Autodesk Fusion 360 part; units mm, degrees
(part 2 of 2)
  arc A221 (-17.6971, -6.491) -> (-17.5951, -6.2945) centre (-17.5563, -6.4394) cw
  arc A222 (-18.1326, 5.1508) -> (-17.9345, 5.2498) centre (-17.9883, 5.1098) cw
  arc A223 (-17.4949, -7.0179) -> (-17.6971, -6.491) centre (0, 0) cw
  arc A224 (-15.4345, -10.5349) -> (-15.6535, -10.5019) centre (-15.5289, -10.4184) cw
  arc A225 (-17.2875, 7.0957) -> (-16.8407, 8.0992) centre (-17.0376, 7.5856) ccw
  arc A226 (-16.9217, 8.3053) -> (-16.6655, 8.8082) centre (0, 0) cw
  arc A227 (-18.1566, -4.4208) -> (-18.385, -3.3464) centre (-18.2425, -3.8776) ccw
  arc A228 (-18.8368, -0.7046) -> (-18.679, -0.5492) centre (-18.6869, -0.699) cw
  arc A229 (-17.5951, 6.2945) -> (-17.6971, 6.491) centre (-17.5563, 6.4394) cw
  arc A230 (-17.9345, -5.2498) -> (-18.1326, -5.1508) centre (-17.9883, -5.1098) cw
  arc A231 (-18.1566, 4.4208) -> (-18.2787, 4.6056) centre (-18.1332, 4.569) cw
  arc A232 (-17.4949, 7.0179) -> (-17.2875, 7.0957) centre (-17.3557, 6.9621) cw
  arc A233 (-18.679, -0.5492) -> (-18.679, 0.5492) centre (-18.65, 0) ccw
  arc A234 (-14.2487, -12.0905) -> (-14.47, -12.0807) centre (-14.3548, -11.9845) cw
  arc A235 (-18.66, 2.6698) -> (-18.5717, 3.2272) centre (0, 0) cw
  arc A236 (-15.4345, 10.5349) -> (-14.7888, 11.4236) centre (-15.0882, 10.9622) ccw
  arc A237 (-15.9609, 10.0286) -> (-15.6535, 10.5019) centre (0, 0) cw
  arc A238 (-14.7888, 11.4236) -> (-14.8251, 11.6421) centre (-14.7072, 11.5494) cw
  arc A239 (-14.47, 12.0807) -> (-14.2487, 12.0905) centre (-14.3548, 11.9845) cw
  circle A240 centre (0, 0) radius 19
extrude "Extrude2" add sketch "60t gt2" along normal blind 7 contours A0 A1 A2 A3 A4 A5 A6 A7 A8 A9 A10 A11 A12 A13 A14 A15 A16 A17 A18 A19 A20 A21 A22 A23 A24 A25 A26 A27 A28 A29 A30 A31 A32 A33 A34 A35 A36 A37 A38 A39 A40 A41 A42 A43 A44 A45 A46 A47 A48 A49 A50 A51 A52 A53 A54 A55 A56 A57 A58 A59 A60 A61 A62 A63 A64 A65 A66 A67 A68 A69 A70 A71 A72 A73 A74 A75 A76 A77 A78 A79 A80 A81 A82 A83 A84 A85 A86 A87 A88 A89 A90 A91 A92 A93 A94 A95 A96 A97 A98 A99 A100 A101 A102 A103 A104 A105 A106 A107 A108 A109 A110 A111 A112 A113 A114 A115 A116 A117 A118 A119 A120 A121 A122 A123 A124 A125 A126 A127 A128 A129 A130 A131 A132 A133 A134 A135 A136 A137 A138 A139 A140 A141 A142 A143 A144 A145 A146 A147 A148 A149 A150 A151 A152 A153 A154 A155 A156 A157 A158 A159 A160 A161 A162 A163 A164 A165 A166 A167 A168 A169 A170 A171 A172 A173 A174 A175 A176 A177 A178 A179 A180 A181 A182 A183 A184 A185 A186 A187 A188 A189 A190 A191 A192 A193 A194 A195 A196 A197 A198 A199 A200 A201 A202 A203 A204 A205 A206 A207 A208 A209 A210 A211 A212 A213 A214 A215 A216 A217 A218 A219 A220 A221 A222 A223 A224 A225 A226 A227 A228 A229 A230 A231 A232 A233 A234 A235 A236 A237 A238 A239
sketch "Sketch8" plane through (0, 0, 0) normal (0, 0, -1) x (1, 0, 0)
  circle A0 centre (0, 0) radius 20
  arc A1 (-14.8251, -11.6421) -> (-14.47, -12.0807) centre (0, 0) ccw
  arc A2 (-14.47, -12.0807) -> (-14.2487, -12.0905) centre (-14.3548, -11.9845) ccw
  arc A3 (-13.5137, -12.9069) -> (-14.2487, -12.0905) centre (-13.8597, -12.4793) ccw
  arc A4 (-13.5137, -12.9069) -> (-13.527, -13.1279) centre (-13.4194, -13.0235) ccw
  arc A5 (-13.527, -13.1279) -> (-13.1279, -13.527) centre (0, 0) ccw
  arc A6 (-13.1279, -13.527) -> (-12.9069, -13.5137) centre (-13.0235, -13.4194) ccw
  arc A7 (-12.0905, -14.2487) -> (-12.9069, -13.5137) centre (-12.4793, -13.8597) ccw
  arc A8 (-12.0905, -14.2487) -> (-12.0807, -14.47) centre (-11.9845, -14.3548) ccw
  arc A9 (-12.0807, -14.47) -> (-11.6421, -14.8251) centre (0, 0) ccw
  arc A10 (-11.6421, -14.8251) -> (-11.4236, -14.7888) centre (-11.5494, -14.7072) ccw
  arc A11 (-10.5349, -15.4345) -> (-11.4236, -14.7888) centre (-10.9622, -15.0882) ccw
  arc A12 (-10.5349, -15.4345) -> (-10.5019, -15.6535) centre (-10.4184, -15.5289) ccw
  arc A13 (-10.5019, -15.6535) -> (-10.0286, -15.9609) centre (0, 0) ccw
  arc A14 (-10.0286, -15.9609) -> (-9.8152, -15.9019) centre (-9.9488, -15.8338) ccw
  arc A15 (-8.8639, -16.4511) -> (-9.8152, -15.9019) centre (-9.325, -16.1514) ccw
  arc A16 (-8.8639, -16.4511) -> (-8.8082, -16.6655) centre (-8.7381, -16.5329) ccw
  arc A17 (-8.8082, -16.6655) -> (-8.3053, -16.9217) centre (0, 0) ccw
  arc A18 (-8.3053, -16.9217) -> (-8.0992, -16.8407) centre (-8.2393, -16.787) ccw
  arc A19 (-7.0957, -17.2875) -> (-8.0992, -16.8407) centre (-7.5856, -17.0376) ccw
  arc A20 (-7.0957, -17.2875) -> (-7.0179, -17.4949) centre (-6.9621, -17.3557) ccw
  arc A21 (-7.0179, -17.4949) -> (-6.491, -17.6971) centre (0, 0) ccw
  arc A22 (-6.491, -17.6971) -> (-6.2945, -17.5951) centre (-6.4394, -17.5563) ccw
  arc A23 (-5.2498, -17.9345) -> (-6.2945, -17.5951) centre (-5.7632, -17.7372) ccw
  arc A24 (-5.2498, -17.9345) -> (-5.1508, -18.1326) centre (-5.1098, -17.9883) ccw
  arc A25 (-5.1508, -18.1326) -> (-4.6056, -18.2787) centre (0, 0) ccw
  arc A26 (-4.6056, -18.2787) -> (-4.4208, -18.1566) centre (-4.569, -18.1332) ccw
  arc A27 (-3.3464, -18.385) -> (-4.4208, -18.1566) centre (-3.8776, -18.2425) ccw
  arc A28 (-3.3464, -18.385) -> (-3.2272, -18.5717) centre (-3.2015, -18.4239) ccw
  arc A29 (-3.2272, -18.5717) -> (-2.6698, -18.66) centre (0, 0) ccw
  arc A30 (-2.6698, -18.66) -> (-2.4987, -18.5193) centre (-2.6485, -18.5115) ccw
  arc A31 (-1.4063, -18.6341) -> (-2.4987, -18.5193) centre (-1.9495, -18.5478) ccw
  arc A32 (-1.4063, -18.6341) -> (-1.2682, -18.8073) centre (-1.2581, -18.6576) ccw
  arc A33 (-1.2682, -18.8073) -> (-0.7046, -18.8368) centre (0, 0) ccw
  arc A34 (-0.7046, -18.8368) -> (-0.5492, -18.679) centre (-0.699, -18.6869) ccw
  arc A35 (0.5492, -18.679) -> (-0.5492, -18.679) centre (0, -18.65) ccw
  arc A36 (0.5492, -18.679) -> (0.7046, -18.8368) centre (0.699, -18.6869) ccw
  arc A37 (0.7046, -18.8368) -> (1.2682, -18.8073) centre (0, 0) ccw
  arc A38 (1.2682, -18.8073) -> (1.4063, -18.6341) centre (1.2581, -18.6576) ccw
  arc A39 (2.4987, -18.5193) -> (1.4063, -18.6341) centre (1.9495, -18.5478) ccw
  arc A40 (2.4987, -18.5193) -> (2.6698, -18.66) centre (2.6485, -18.5115) ccw
  arc A41 (2.6698, -18.66) -> (3.2272, -18.5717) centre (0, 0) ccw
  arc A42 (3.2272, -18.5717) -> (3.3464, -18.385) centre (3.2015, -18.4239) ccw
  arc A43 (4.4208, -18.1566) -> (3.3464, -18.385) centre (3.8776, -18.2425) ccw
  arc A44 (4.4208, -18.1566) -> (4.6056, -18.2787) centre (4.569, -18.1332) ccw
  arc A45 (4.6056, -18.2787) -> (5.1508, -18.1326) centre (0, 0) ccw
  arc A46 (5.1508, -18.1326) -> (5.2498, -17.9345) centre (5.1098, -17.9883) ccw
  arc A47 (6.2945, -17.5951) -> (5.2498, -17.9345) centre (5.7632, -17.7372) ccw
  arc A48 (6.2945, -17.5951) -> (6.491, -17.6971) centre (6.4394, -17.5563) ccw
  arc A49 (6.491, -17.6971) -> (7.0179, -17.4949) centre (0, 0) ccw
  arc A50 (7.0179, -17.4949) -> (7.0957, -17.2875) centre (6.9621, -17.3557) ccw
  arc A51 (8.0992, -16.8407) -> (7.0957, -17.2875) centre (7.5856, -17.0376) ccw
  arc A52 (8.0992, -16.8407) -> (8.3053, -16.9217) centre (8.2393, -16.787) ccw
  arc A53 (8.3053, -16.9217) -> (8.8082, -16.6655) centre (0, 0) ccw
  arc A54 (8.8082, -16.6655) -> (8.8639, -16.4511) centre (8.7381, -16.5329) ccw
  arc A55 (9.8152, -15.9019) -> (8.8639, -16.4511) centre (9.325, -16.1514) ccw
  arc A56 (9.8152, -15.9019) -> (10.0286, -15.9609) centre (9.9488, -15.8338) ccw
  arc A57 (10.0286, -15.9609) -> (10.5019, -15.6535) centre (0, 0) ccw
  arc A58 (10.5019, -15.6535) -> (10.5349, -15.4345) centre (10.4184, -15.5289) ccw
  arc A59 (11.4236, -14.7888) -> (10.5349, -15.4345) centre (10.9622, -15.0882) ccw
  arc A60 (11.4236, -14.7888) -> (11.6421, -14.8251) centre (11.5494, -14.7072) ccw
  arc A61 (11.6421, -14.8251) -> (12.0807, -14.47) centre (0, 0) ccw
  arc A62 (12.0807, -14.47) -> (12.0905, -14.2487) centre (11.9845, -14.3548) ccw
  arc A63 (12.9069, -13.5137) -> (12.0905, -14.2487) centre (12.4793, -13.8597) ccw
  arc A64 (12.9069, -13.5137) -> (13.1279, -13.527) centre (13.0235, -13.4194) ccw
  arc A65 (13.1279, -13.527) -> (13.527, -13.1279) centre (0, 0) ccw
  arc A66 (13.527, -13.1279) -> (13.5137, -12.9069) centre (13.4194, -13.0235) ccw
  arc A67 (14.2487, -12.0905) -> (13.5137, -12.9069) centre (13.8597, -12.4793) ccw
  arc A68 (14.2487, -12.0905) -> (14.47, -12.0807) centre (14.3548, -11.9845) ccw
  arc A69 (14.47, -12.0807) -> (14.8251, -11.6421) centre (0, 0) ccw
  arc A70 (14.8251, -11.6421) -> (14.7888, -11.4236) centre (14.7072, -11.5494) ccw
  arc A71 (15.4345, -10.5349) -> (14.7888, -11.4236) centre (15.0882, -10.9622) ccw
  arc A72 (15.4345, -10.5349) -> (15.6535, -10.5019) centre (15.5289, -10.4184) ccw
  arc A73 (15.6535, -10.5019) -> (15.9609, -10.0286) centre (0, 0) ccw
  arc A74 (15.9609, -10.0286) -> (15.9019, -9.8152) centre (15.8338, -9.9488) ccw
  arc A75 (16.4511, -8.8639) -> (15.9019, -9.8152) centre (16.1514, -9.325) ccw
  arc A76 (16.4511, -8.8639) -> (16.6655, -8.8082) centre (16.5329, -8.7381) ccw
  arc A77 (16.6655, -8.8082) -> (16.9217, -8.3053) centre (0, 0) ccw
  arc A78 (16.9217, -8.3053) -> (16.8407, -8.0992) centre (16.787, -8.2393) ccw
  arc A79 (17.2875, -7.0957) -> (16.8407, -8.0992) centre (17.0376, -7.5856) ccw
  arc A80 (17.2875, -7.0957) -> (17.4949, -7.0179) centre (17.3557, -6.9621) ccw
  arc A81 (17.4949, -7.0179) -> (17.6971, -6.491) centre (0, 0) ccw
  arc A82 (17.6971, -6.491) -> (17.5951, -6.2945) centre (17.5563, -6.4394) ccw
  arc A83 (17.9345, -5.2498) -> (17.5951, -6.2945) centre (17.7372, -5.7632) ccw
  arc A84 (17.9345, -5.2498) -> (18.1326, -5.1508) centre (17.9883, -5.1098) ccw
  arc A85 (18.1326, -5.1508) -> (18.2787, -4.6056) centre (0, 0) ccw
  arc A86 (18.2787, -4.6056) -> (18.1566, -4.4208) centre (18.1332, -4.569) ccw
  arc A87 (18.385, -3.3464) -> (18.1566, -4.4208) centre (18.2425, -3.8776) ccw
  arc A88 (18.385, -3.3464) -> (18.5717, -3.2272) centre (18.4239, -3.2015) ccw
  arc A89 (18.5717, -3.2272) -> (18.66, -2.6698) centre (0, 0) ccw
  arc A90 (18.66, -2.6698) -> (18.5193, -2.4987) centre (18.5115, -2.6485) ccw
  arc A91 (18.6341, -1.4063) -> (18.5193, -2.4987) centre (18.5478, -1.9495) ccw
  arc A92 (18.6341, -1.4063) -> (18.8073, -1.2682) centre (18.6576, -1.2581) ccw
  arc A93 (18.8073, -1.2682) -> (18.8368, -0.7046) centre (0, 0) ccw
  arc A94 (18.8368, -0.7046) -> (18.679, -0.5492) centre (18.6869, -0.699) ccw
  arc A95 (18.679, 0.5492) -> (18.679, -0.5492) centre (18.65, 0) ccw
  arc A96 (18.679, 0.5492) -> (18.8368, 0.7046) centre (18.6869, 0.699) ccw
  arc A97 (18.8368, 0.7046) -> (18.8073, 1.2682) centre (0, 0) ccw
  arc A98 (18.8073, 1.2682) -> (18.6341, 1.4063) centre (18.6576, 1.2581) ccw
  arc A99 (18.5193, 2.4987) -> (18.6341, 1.4063) centre (18.5478, 1.9495) ccw
  arc A100 (18.5193, 2.4987) -> (18.66, 2.6698) centre (18.5115, 2.6485) ccw
  arc A101 (18.66, 2.6698) -> (18.5717, 3.2272) centre (0, 0) ccw
  arc A102 (18.5717, 3.2272) -> (18.385, 3.3464) centre (18.4239, 3.2015) ccw
  arc A103 (18.1566, 4.4208) -> (18.385, 3.3464) centre (18.2425, 3.8776) ccw
  arc A104 (18.1566, 4.4208) -> (18.2787, 4.6056) centre (18.1332, 4.569) ccw
  arc A105 (18.2787, 4.6056) -> (18.1326, 5.1508) centre (0, 0) ccw
  arc A106 (18.1326, 5.1508) -> (17.9345, 5.2498) centre (17.9883, 5.1098) ccw
  arc A107 (17.5951, 6.2945) -> (17.9345, 5.2498) centre (17.7372, 5.7632) ccw
  arc A108 (17.5951, 6.2945) -> (17.6971, 6.491) centre (17.5563, 6.4394) ccw
  arc A109 (17.6971, 6.491) -> (17.4949, 7.0179) centre (0, 0) ccw
  arc A110 (17.4949, 7.0179) -> (17.2875, 7.0957) centre (17.3557, 6.9621) ccw
  arc A111 (16.8407, 8.0992) -> (17.2875, 7.0957) centre (17.0376, 7.5856) ccw
  arc A112 (16.8407, 8.0992) -> (16.9217, 8.3053) centre (16.787, 8.2393) ccw
  arc A113 (16.9217, 8.3053) -> (16.6655, 8.8082) centre (0, 0) ccw
  arc A114 (16.6655, 8.8082) -> (16.4511, 8.8639) centre (16.5329, 8.7381) ccw
  arc A115 (15.9019, 9.8152) -> (16.4511, 8.8639) centre (16.1514, 9.325) ccw
  arc A116 (15.9019, 9.8152) -> (15.9609, 10.0286) centre (15.8338, 9.9488) ccw
  arc A117 (15.9609, 10.0286) -> (15.6535, 10.5019) centre (0, 0) ccw
  arc A118 (15.6535, 10.5019) -> (15.4345, 10.5349) centre (15.5289, 10.4184) ccw
  arc A119 (14.7888, 11.4236) -> (15.4345, 10.5349) centre (15.0882, 10.9622) ccw
  arc A120 (14.7888, 11.4236) -> (14.8251, 11.6421) centre (14.7072, 11.5494) ccw
  arc A121 (14.8251, 11.6421) -> (14.47, 12.0807) centre (0, 0) ccw
  arc A122 (14.47, 12.0807) -> (14.2487, 12.0905) centre (14.3548, 11.9845) ccw
  arc A123 (13.5137, 12.9069) -> (14.2487, 12.0905) centre (13.8597, 12.4793) ccw
  arc A124 (13.5137, 12.9069) -> (13.527, 13.1279) centre (13.4194, 13.0235) ccw
  arc A125 (13.527, 13.1279) -> (13.1279, 13.527) centre (0, 0) ccw
  arc A126 (13.1279, 13.527) -> (12.9069, 13.5137) centre (13.0235, 13.4194) ccw
  arc A127 (12.0905, 14.2487) -> (12.9069, 13.5137) centre (12.4793, 13.8597) ccw
  arc A128 (12.0905, 14.2487) -> (12.0807, 14.47) centre (11.9845, 14.3548) ccw
  arc A129 (12.0807, 14.47) -> (11.6421, 14.8251) centre (0, 0) ccw
  arc A130 (11.6421, 14.8251) -> (11.4236, 14.7888) centre (11.5494, 14.7072) ccw
  arc A131 (10.5349, 15.4345) -> (11.4236, 14.7888) centre (10.9622, 15.0882) ccw
  arc A132 (10.5349, 15.4345) -> (10.5019, 15.6535) centre (10.4184, 15.5289) ccw
  arc A133 (10.5019, 15.6535) -> (10.0286, 15.9609) centre (0, 0) ccw
  arc A134 (10.0286, 15.9609) -> (9.8152, 15.9019) centre (9.9488, 15.8338) ccw
  arc A135 (8.8639, 16.4511) -> (9.8152, 15.9019) centre (9.325, 16.1514) ccw
  arc A136 (8.8639, 16.4511) -> (8.8082, 16.6655) centre (8.7381, 16.5329) ccw
  arc A137 (8.8082, 16.6655) -> (8.3053, 16.9217) centre (0, 0) ccw
  arc A138 (8.3053, 16.9217) -> (8.0992, 16.8407) centre (8.2393, 16.787) ccw
  arc A139 (7.0957, 17.2875) -> (8.0992, 16.8407) centre (7.5856, 17.0376) ccw
  arc A140 (7.0957, 17.2875) -> (7.0179, 17.4949) centre (6.9621, 17.3557) ccw
  arc A141 (7.0179, 17.4949) -> (6.491, 17.6971) centre (0, 0) ccw
  arc A142 (6.491, 17.6971) -> (6.2945, 17.5951) centre (6.4394, 17.5563) ccw
  arc A143 (5.2498, 17.9345) -> (6.2945, 17.5951) centre (5.7632, 17.7372) ccw
  arc A144 (5.2498, 17.9345) -> (5.1508, 18.1326) centre (5.1098, 17.9883) ccw
  arc A145 (5.1508, 18.1326) -> (4.6056, 18.2787) centre (0, 0) ccw
  arc A146 (4.6056, 18.2787) -> (4.4208, 18.1566) centre (4.569, 18.1332) ccw
  arc A147 (3.3464, 18.385) -> (4.4208, 18.1566) centre (3.8776, 18.2425) ccw
  arc A148 (3.3464, 18.385) -> (3.2272, 18.5717) centre (3.2015, 18.4239) ccw
  arc A149 (3.2272, 18.5717) -> (2.6698, 18.66) centre (0, 0) ccw
  arc A150 (2.6698, 18.66) -> (2.4987, 18.5193) centre (2.6485, 18.5115) ccw
  arc A151 (1.4063, 18.6341) -> (2.4987, 18.5193) centre (1.9495, 18.5478) ccw
  arc A152 (1.4063, 18.6341) -> (1.2682, 18.8073) centre (1.2581, 18.6576) ccw
  arc A153 (1.2682, 18.8073) -> (0.7046, 18.8368) centre (0, 0) ccw
  arc A154 (0.7046, 18.8368) -> (0.5492, 18.679) centre (0.699, 18.6869) ccw
  arc A155 (-0.5492, 18.679) -> (0.5492, 18.679) centre (0, 18.65) ccw
  arc A156 (-0.5492, 18.679) -> (-0.7046, 18.8368) centre (-0.699, 18.6869) ccw
  arc A157 (-0.7046, 18.8368) -> (-1.2682, 18.8073) centre (0, 0) ccw
  arc A158 (-1.2682, 18.8073) -> (-1.4063, 18.6341) centre (-1.2581, 18.6576) ccw
  arc A159 (-2.4987, 18.5193) -> (-1.4063, 18.6341) centre (-1.9495, 18.5478) ccw
  arc A160 (-2.4987, 18.5193) -> (-2.6698, 18.66) centre (-2.6485, 18.5115) ccw
  arc A161 (-2.6698, 18.66) -> (-3.2272, 18.5717) centre (0, 0) ccw
  arc A162 (-3.2272, 18.5717) -> (-3.3464, 18.385) centre (-3.2015, 18.4239) ccw
  arc A163 (-4.4208, 18.1566) -> (-3.3464, 18.385) centre (-3.8776, 18.2425) ccw
  arc A164 (-4.4208, 18.1566) -> (-4.6056, 18.2787) centre (-4.569, 18.1332) ccw
  arc A165 (-4.6056, 18.2787) -> (-5.1508, 18.1326) centre (0, 0) ccw
  arc A166 (-5.1508, 18.1326) -> (-5.2498, 17.9345) centre (-5.1098, 17.9883) ccw
  arc A167 (-6.2945, 17.5951) -> (-5.2498, 17.9345) centre (-5.7632, 17.7372) ccw
  arc A168 (-6.2945, 17.5951) -> (-6.491, 17.6971) centre (-6.4394, 17.5563) ccw
  arc A169 (-6.491, 17.6971) -> (-7.0179, 17.4949) centre (0, 0) ccw
  arc A170 (-7.0179, 17.4949) -> (-7.0957, 17.2875) centre (-6.9621, 17.3557) ccw
  arc A171 (-8.0992, 16.8407) -> (-7.0957, 17.2875) centre (-7.5856, 17.0376) ccw
  arc A172 (-8.0992, 16.8407) -> (-8.3053, 16.9217) centre (-8.2393, 16.787) ccw
  arc A173 (-8.3053, 16.9217) -> (-8.8082, 16.6655) centre (0, 0) ccw
  arc A174 (-8.8082, 16.6655) -> (-8.8639, 16.4511) centre (-8.7381, 16.5329) ccw
  arc A175 (-9.8152, 15.9019) -> (-8.8639, 16.4511) centre (-9.325, 16.1514) ccw
  arc A176 (-9.8152, 15.9019) -> (-10.0286, 15.9609) centre (-9.9488, 15.8338) ccw
  arc A177 (-10.0286, 15.9609) -> (-10.5019, 15.6535) centre (0, 0) ccw
  arc A178 (-10.5019, 15.6535) -> (-10.5349, 15.4345) centre (-10.4184, 15.5289) ccw
  arc A179 (-11.4236, 14.7888) -> (-10.5349, 15.4345) centre (-10.9622, 15.0882) ccw
  arc A180 (-11.4236, 14.7888) -> (-11.6421, 14.8251) centre (-11.5494, 14.7072) ccw
  arc A181 (-11.6421, 14.8251) -> (-12.0807, 14.47) centre (0, 0) ccw
  arc A182 (-12.0807, 14.47) -> (-12.0905, 14.2487) centre (-11.9845, 14.3548) ccw
  arc A183 (-12.9069, 13.5137) -> (-12.0905, 14.2487) centre (-12.4793, 13.8597) ccw
  arc A184 (-12.9069, 13.5137) -> (-13.1279, 13.527) centre (-13.0235, 13.4194) ccw
  arc A185 (-13.1279, 13.527) -> (-13.527, 13.1279) centre (0, 0) ccw
  arc A186 (-13.527, 13.1279) -> (-13.5137, 12.9069) centre (-13.4194, 13.0235) ccw
  arc A187 (-14.2487, 12.0905) -> (-13.5137, 12.9069) centre (-13.8597, 12.4793) ccw
  arc A188 (-14.2487, 12.0905) -> (-14.47, 12.0807) centre (-14.3548, 11.9845) ccw
  arc A189 (-14.47, 12.0807) -> (-14.8251, 11.6421) centre (0, 0) ccw
  arc A190 (-14.8251, 11.6421) -> (-14.7888, 11.4236) centre (-14.7072, 11.5494) ccw
  arc A191 (-15.4345, 10.5349) -> (-14.7888, 11.4236) centre (-15.0882, 10.9622) ccw
  arc A192 (-15.4345, 10.5349) -> (-15.6535, 10.5019) centre (-15.5289, 10.4184) ccw
  arc A193 (-15.6535, 10.5019) -> (-15.9609, 10.0286) centre (0, 0) ccw
  arc A194 (-15.9609, 10.0286) -> (-15.9019, 9.8152) centre (-15.8338, 9.9488) ccw
  arc A195 (-16.4511, 8.8639) -> (-15.9019, 9.8152) centre (-16.1514, 9.325) ccw
  arc A196 (-16.4511, 8.8639) -> (-16.6655, 8.8082) centre (-16.5329, 8.7381) ccw
  arc A197 (-16.6655, 8.8082) -> (-16.9217, 8.3053) centre (0, 0) ccw
  arc A198 (-16.9217, 8.3053) -> (-16.8407, 8.0992) centre (-16.787, 8.2393) ccw
  arc A199 (-17.2875, 7.0957) -> (-16.8407, 8.0992) centre (-17.0376, 7.5856) ccw
  arc A200 (-17.2875, 7.0957) -> (-17.4949, 7.0179) centre (-17.3557, 6.9621) ccw
  arc A201 (-17.4949, 7.0179) -> (-17.6971, 6.491) centre (0, 0) ccw
  arc A202 (-17.6971, 6.491) -> (-17.5951, 6.2945) centre (-17.5563, 6.4394) ccw
  arc A203 (-17.9345, 5.2498) -> (-17.5951, 6.2945) centre (-17.7372, 5.7632) ccw
  arc A204 (-17.9345, 5.2498) -> (-18.1326, 5.1508) centre (-17.9883, 5.1098) ccw
  arc A205 (-18.1326, 5.1508) -> (-18.2787, 4.6056) centre (0, 0) ccw
  arc A206 (-18.2787, 4.6056) -> (-18.1566, 4.4208) centre (-18.1332, 4.569) ccw
  arc A207 (-18.385, 3.3464) -> (-18.1566, 4.4208) centre (-18.2425, 3.8776) ccw
  arc A208 (-18.385, 3.3464) -> (-18.5717, 3.2272) centre (-18.4239, 3.2015) ccw
  arc A209 (-18.5717, 3.2272) -> (-18.66, 2.6698) centre (0, 0) ccw
  arc A210 (-18.66, 2.6698) -> (-18.5193, 2.4987) centre (-18.5115, 2.6485) ccw
  arc A211 (-18.6341, 1.4063) -> (-18.5193, 2.4987) centre (-18.5478, 1.9495) ccw
  arc A212 (-18.6341, 1.4063) -> (-18.8073, 1.2682) centre (-18.6576, 1.2581) ccw
  arc A213 (-18.8073, 1.2682) -> (-18.8368, 0.7046) centre (0, 0) ccw
  arc A214 (-18.8368, 0.7046) -> (-18.679, 0.5492) centre (-18.6869, 0.699) ccw
  arc A215 (-18.679, -0.5492) -> (-18.679, 0.5492) centre (-18.65, 0) ccw
  arc A216 (-18.679, -0.5492) -> (-18.8368, -0.7046) centre (-18.6869, -0.699) ccw
  arc A217 (-18.8368, -0.7046) -> (-18.8073, -1.2682) centre (0, 0) ccw
  arc A218 (-18.8073, -1.2682) -> (-18.6341, -1.4063) centre (-18.6576, -1.2581) ccw
  arc A219 (-18.5193, -2.4987) -> (-18.6341, -1.4063) centre (-18.5478, -1.9495) ccw
  arc A220 (-18.5193, -2.4987) -> (-18.66, -2.6698) centre (-18.5115, -2.6485) ccw
  arc A221 (-18.66, -2.6698) -> (-18.5717, -3.2272) centre (0, 0) ccw
  arc A222 (-18.5717, -3.2272) -> (-18.385, -3.3464) centre (-18.4239, -3.2015) ccw
  arc A223 (-18.1566, -4.4208) -> (-18.385, -3.3464) centre (-18.2425, -3.8776) ccw
  arc A224 (-18.1566, -4.4208) -> (-18.2787, -4.6056) centre (-18.1332, -4.569) ccw
  arc A225 (-18.2787, -4.6056) -> (-18.1326, -5.1508) centre (0, 0) ccw
  arc A226 (-18.1326, -5.1508) -> (-17.9345, -5.2498) centre (-17.9883, -5.1098) ccw
  arc A227 (-17.5951, -6.2945) -> (-17.9345, -5.2498) centre (-17.7372, -5.7632) ccw
  arc A228 (-17.5951, -6.2945) -> (-17.6971, -6.491) centre (-17.5563, -6.4394) ccw
  arc A229 (-17.6971, -6.491) -> (-17.4949, -7.0179) centre (0, 0) ccw
  arc A230 (-17.4949, -7.0179) -> (-17.2875, -7.0957) centre (-17.3557, -6.9621) ccw
  arc A231 (-16.8407, -8.0992) -> (-17.2875, -7.0957) centre (-17.0376, -7.5856) ccw
  arc A232 (-16.8407, -8.0992) -> (-16.9217, -8.3053) centre (-16.787, -8.2393) ccw
  arc A233 (-16.9217, -8.3053) -> (-16.6655, -8.8082) centre (0, 0) ccw
  arc A234 (-16.6655, -8.8082) -> (-16.4511, -8.8639) centre (-16.5329, -8.7381) ccw
  arc A235 (-15.9019, -9.8152) -> (-16.4511, -8.8639) centre (-16.1514, -9.325) ccw
  arc A236 (-15.9019, -9.8152) -> (-15.9609, -10.0286) centre (-15.8338, -9.9488) ccw
  arc A237 (-15.9609, -10.0286) -> (-15.6535, -10.5019) centre (0, 0) ccw
  arc A238 (-15.6535, -10.5019) -> (-15.4345, -10.5349) centre (-15.5289, -10.4184) ccw
  arc A239 (-14.7888, -11.4236) -> (-15.4345, -10.5349) centre (-15.0882, -10.9622) ccw
  arc A240 (-14.7888, -11.4236) -> (-14.8251, -11.6421) centre (-14.7072, -11.5494) ccw
  dimension "d55" = 40
  constraint coincident A0.centre A1.centre
  measures "d55" diameter of A0
extrude "Extrude9" add sketch "Sketch8" along normal blind 1 contours A0 | A1 A2 A3 A4 A5 A6 A7 A8 A9 A10 A11 A12 A13 A14 A15 A16 A17 A18 A19 A20 A21 A22 A23 A24 A25 A26 A27 A28 A29 A30 A31 A32 A33 A34 A35 A36 A37 A38 A39 A40 A41 A42 A43 A44 A45 A46 A47 A48 A49 A50 A51 A52 A53 A54 A55 A56 A57 A58 A59 A60 A61 A62 A63 A64 A65 A66 A67 A68 A69 A70 A71 A72 A73 A74 A75 A76 A77 A78 A79 A80 A81 A82 A83 A84 A85 A86 A87 A88 A89 A90 A91 A92 A93 A94 A95 A96 A97 A98 A99 A100 A101 A102 A103 A104 A105 A106 A107 A108 A109 A110 A111 A112 A113 A114 A115 A116 A117 A118 A119 A120 A121 A122 A123 A124 A125 A126 A127 A128 A129 A130 A131 A132 A133 A134 A135 A136 A137 A138 A139 A140 A141 A142 A143 A144 A145 A146 A147 A148 A149 A150 A151 A152 A153 A154 A155 A156 A157 A158 A159 A160 A161 A162 A163 A164 A165 A166 A167 A168 A169 A170 A171 A172 A173 A174 A175 A176 A177 A178 A179 A180 A181 A182 A183 A184 A185 A186 A187 A188 A189 A190 A191 A192 A193 A194 A195 A196 A197 A198 A199 A200 A201 A202 A203 A204 A205 A206 A207 A208 A209 A210 A211 A212 A213 A214 A215 A216 A217 A218 A219 A220 A221 A222 A223 A224 A225 A226 A227 A228 A229 A230 A231 A232 A233 A234 A235 A236 A237 A238 A239 A240
sketch "Sketch9" plane through (0, 0, 7) normal (0, 0, 1) x (-1, 0, 0)
  circle A0 centre (0, 0) radius 20
  arc A1 (14.47, -12.0807) -> (14.8251, -11.6421) centre (0, 0) ccw
  arc A2 (14.8251, -11.6421) -> (14.7888, -11.4236) centre (14.7072, -11.5494) ccw
  arc A3 (15.4345, -10.5349) -> (14.7888, -11.4236) centre (15.0882, -10.9622) ccw
  arc A4 (15.4345, -10.5349) -> (15.6535, -10.5019) centre (15.5289, -10.4184) ccw
  arc A5 (15.6535, -10.5019) -> (15.9609, -10.0286) centre (0, 0) ccw
  arc A6 (15.9609, -10.0286) -> (15.9019, -9.8152) centre (15.8338, -9.9488) ccw
  arc A7 (16.4511, -8.8639) -> (15.9019, -9.8152) centre (16.1514, -9.325) ccw
  arc A8 (16.4511, -8.8639) -> (16.6655, -8.8082) centre (16.5329, -8.7381) ccw
  arc A9 (16.6655, -8.8082) -> (16.9217, -8.3053) centre (0, 0) ccw
  arc A10 (16.9217, -8.3053) -> (16.8407, -8.0992) centre (16.787, -8.2393) ccw
  arc A11 (17.2875, -7.0957) -> (16.8407, -8.0992) centre (17.0376, -7.5856) ccw
  arc A12 (17.2875, -7.0957) -> (17.4949, -7.0179) centre (17.3557, -6.9621) ccw
  arc A13 (17.4949, -7.0179) -> (17.6971, -6.491) centre (0, 0) ccw
  arc A14 (17.6971, -6.491) -> (17.5951, -6.2945) centre (17.5563, -6.4394) ccw
  arc A15 (17.9345, -5.2498) -> (17.5951, -6.2945) centre (17.7372, -5.7632) ccw
  arc A16 (17.9345, -5.2498) -> (18.1326, -5.1508) centre (17.9883, -5.1098) ccw
  arc A17 (18.1326, -5.1508) -> (18.2787, -4.6056) centre (0, 0) ccw
  arc A18 (18.2787, -4.6056) -> (18.1566, -4.4208) centre (18.1332, -4.569) ccw
  arc A19 (18.385, -3.3464) -> (18.1566, -4.4208) centre (18.2425, -3.8776) ccw
  arc A20 (18.385, -3.3464) -> (18.5717, -3.2272) centre (18.4239, -3.2015) ccw
  arc A21 (18.5717, -3.2272) -> (18.66, -2.6698) centre (0, 0) ccw
  arc A22 (18.66, -2.6698) -> (18.5193, -2.4987) centre (18.5115, -2.6485) ccw
  arc A23 (18.6341, -1.4063) -> (18.5193, -2.4987) centre (18.5478, -1.9495) ccw
  arc A24 (18.6341, -1.4063) -> (18.8073, -1.2682) centre (18.6576, -1.2581) ccw
  arc A25 (18.8073, -1.2682) -> (18.8368, -0.7046) centre (0, 0) ccw
  arc A26 (18.8368, -0.7046) -> (18.679, -0.5492) centre (18.6869, -0.699) ccw
  arc A27 (18.679, 0.5492) -> (18.679, -0.5492) centre (18.65, 0) ccw
  arc A28 (18.679, 0.5492) -> (18.8368, 0.7046) centre (18.6869, 0.699) ccw
  arc A29 (18.8368, 0.7046) -> (18.8073, 1.2682) centre (0, 0) ccw
  arc A30 (18.8073, 1.2682) -> (18.6341, 1.4063) centre (18.6576, 1.2581) ccw
  arc A31 (18.5193, 2.4987) -> (18.6341, 1.4063) centre (18.5478, 1.9495) ccw
  arc A32 (18.5193, 2.4987) -> (18.66, 2.6698) centre (18.5115, 2.6485) ccw
  arc A33 (18.66, 2.6698) -> (18.5717, 3.2272) centre (0, 0) ccw
  arc A34 (18.5717, 3.2272) -> (18.385, 3.3464) centre (18.4239, 3.2015) ccw
  arc A35 (18.1566, 4.4208) -> (18.385, 3.3464) centre (18.2425, 3.8776) ccw
  arc A36 (18.1566, 4.4208) -> (18.2787, 4.6056) centre (18.1332, 4.569) ccw
  arc A37 (18.2787, 4.6056) -> (18.1326, 5.1508) centre (0, 0) ccw
  arc A38 (18.1326, 5.1508) -> (17.9345, 5.2498) centre (17.9883, 5.1098) ccw
  arc A39 (17.5951, 6.2945) -> (17.9345, 5.2498) centre (17.7372, 5.7632) ccw
  arc A40 (17.5951, 6.2945) -> (17.6971, 6.491) centre (17.5563, 6.4394) ccw
  arc A41 (17.6971, 6.491) -> (17.4949, 7.0179) centre (0, 0) ccw
  arc A42 (17.4949, 7.0179) -> (17.2875, 7.0957) centre (17.3557, 6.9621) ccw
  arc A43 (16.8407, 8.0992) -> (17.2875, 7.0957) centre (17.0376, 7.5856) ccw
  arc A44 (16.8407, 8.0992) -> (16.9217, 8.3053) centre (16.787, 8.2393) ccw
  arc A45 (16.9217, 8.3053) -> (16.6655, 8.8082) centre (0, 0) ccw
  arc A46 (16.6655, 8.8082) -> (16.4511, 8.8639) centre (16.5329, 8.7381) ccw
  arc A47 (15.9019, 9.8152) -> (16.4511, 8.8639) centre (16.1514, 9.325) ccw
  arc A48 (15.9019, 9.8152) -> (15.9609, 10.0286) centre (15.8338, 9.9488) ccw
  arc A49 (15.9609, 10.0286) -> (15.6535, 10.5019) centre (0, 0) ccw
  arc A50 (15.6535, 10.5019) -> (15.4345, 10.5349) centre (15.5289, 10.4184) ccw
  arc A51 (14.7888, 11.4236) -> (15.4345, 10.5349) centre (15.0882, 10.9622) ccw
  arc A52 (14.7888, 11.4236) -> (14.8251, 11.6421) centre (14.7072, 11.5494) ccw
  arc A53 (14.8251, 11.6421) -> (14.47, 12.0807) centre (0, 0) ccw
  arc A54 (14.47, 12.0807) -> (14.2487, 12.0905) centre (14.3548, 11.9845) ccw
  arc A55 (13.5137, 12.9069) -> (14.2487, 12.0905) centre (13.8597, 12.4793) ccw
  arc A56 (13.5137, 12.9069) -> (13.527, 13.1279) centre (13.4194, 13.0235) ccw
  arc A57 (13.527, 13.1279) -> (13.1279, 13.527) centre (0, 0) ccw
  arc A58 (13.1279, 13.527) -> (12.9069, 13.5137) centre (13.0235, 13.4194) ccw
  arc A59 (12.0905, 14.2487) -> (12.9069, 13.5137) centre (12.4793, 13.8597) ccw
  arc A60 (12.0905, 14.2487) -> (12.0807, 14.47) centre (11.9845, 14.3548) ccw
  arc A61 (12.0807, 14.47) -> (11.6421, 14.8251) centre (0, 0) ccw
  arc A62 (11.6421, 14.8251) -> (11.4236, 14.7888) centre (11.5494, 14.7072) ccw
  arc A63 (10.5349, 15.4345) -> (11.4236, 14.7888) centre (10.9622, 15.0882) ccw
  arc A64 (10.5349, 15.4345) -> (10.5019, 15.6535) centre (10.4184, 15.5289) ccw
  arc A65 (10.5019, 15.6535) -> (10.0286, 15.9609) centre (0, 0) ccw
  arc A66 (10.0286, 15.9609) -> (9.8152, 15.9019) centre (9.9488, 15.8338) ccw
  arc A67 (8.8639, 16.4511) -> (9.8152, 15.9019) centre (9.325, 16.1514) ccw
  arc A68 (8.8639, 16.4511) -> (8.8082, 16.6655) centre (8.7381, 16.5329) ccw
  arc A69 (8.8082, 16.6655) -> (8.3053, 16.9217) centre (0, 0) ccw
  arc A70 (8.3053, 16.9217) -> (8.0992, 16.8407) centre (8.2393, 16.787) ccw
  arc A71 (7.0957, 17.2875) -> (8.0992, 16.8407) centre (7.5856, 17.0376) ccw
  arc A72 (7.0957, 17.2875) -> (7.0179, 17.4949) centre (6.9621, 17.3557) ccw
  arc A73 (7.0179, 17.4949) -> (6.491, 17.6971) centre (0, 0) ccw
  arc A74 (6.491, 17.6971) -> (6.2945, 17.5951) centre (6.4394, 17.5563) ccw
  arc A75 (5.2498, 17.9345) -> (6.2945, 17.5951) centre (5.7632, 17.7372) ccw
  arc A76 (5.2498, 17.9345) -> (5.1508, 18.1326) centre (5.1098, 17.9883) ccw
  arc A77 (5.1508, 18.1326) -> (4.6056, 18.2787) centre (0, 0) ccw
  arc A78 (4.6056, 18.2787) -> (4.4208, 18.1566) centre (4.569, 18.1332) ccw
  arc A79 (3.3464, 18.385) -> (4.4208, 18.1566) centre (3.8776, 18.2425) ccw
  arc A80 (3.3464, 18.385) -> (3.2272, 18.5717) centre (3.2015, 18.4239) ccw
  arc A81 (3.2272, 18.5717) -> (2.6698, 18.66) centre (0, 0) ccw
  arc A82 (2.6698, 18.66) -> (2.4987, 18.5193) centre (2.6485, 18.5115) ccw
  arc A83 (1.4063, 18.6341) -> (2.4987, 18.5193) centre (1.9495, 18.5478) ccw
  arc A84 (1.4063, 18.6341) -> (1.2682, 18.8073) centre (1.2581, 18.6576) ccw
  arc A85 (1.2682, 18.8073) -> (0.7046, 18.8368) centre (0, 0) ccw
  arc A86 (0.7046, 18.8368) -> (0.5492, 18.679) centre (0.699, 18.6869) ccw
  arc A87 (-0.5492, 18.679) -> (0.5492, 18.679) centre (0, 18.65) ccw
  arc A88 (-0.5492, 18.679) -> (-0.7046, 18.8368) centre (-0.699, 18.6869) ccw
  arc A89 (-0.7046, 18.8368) -> (-1.2682, 18.8073) centre (0, 0) ccw
  arc A90 (-1.2682, 18.8073) -> (-1.4063, 18.6341) centre (-1.2581, 18.6576) ccw
  arc A91 (-2.4987, 18.5193) -> (-1.4063, 18.6341) centre (-1.9495, 18.5478) ccw
  arc A92 (-2.4987, 18.5193) -> (-2.6698, 18.66) centre (-2.6485, 18.5115) ccw
  arc A93 (-2.6698, 18.66) -> (-3.2272, 18.5717) centre (0, 0) ccw
  arc A94 (-3.2272, 18.5717) -> (-3.3464, 18.385) centre (-3.2015, 18.4239) ccw
  arc A95 (-4.4208, 18.1566) -> (-3.3464, 18.385) centre (-3.8776, 18.2425) ccw
  arc A96 (-4.4208, 18.1566) -> (-4.6056, 18.2787) centre (-4.569, 18.1332) ccw
  arc A97 (-4.6056, 18.2787) -> (-5.1508, 18.1326) centre (0, 0) ccw
  arc A98 (-5.1508, 18.1326) -> (-5.2498, 17.9345) centre (-5.1098, 17.9883) ccw
  arc A99 (-6.2945, 17.5951) -> (-5.2498, 17.9345) centre (-5.7632, 17.7372) ccw
  arc A100 (-6.2945, 17.5951) -> (-6.491, 17.6971) centre (-6.4394, 17.5563) ccw
  arc A101 (-6.491, 17.6971) -> (-7.0179, 17.4949) centre (0, 0) ccw
  arc A102 (-7.0179, 17.4949) -> (-7.0957, 17.2875) centre (-6.9621, 17.3557) ccw
  arc A103 (-8.0992, 16.8407) -> (-7.0957, 17.2875) centre (-7.5856, 17.0376) ccw
  arc A104 (-8.0992, 16.8407) -> (-8.3053, 16.9217) centre (-8.2393, 16.787) ccw
  arc A105 (-8.3053, 16.9217) -> (-8.8082, 16.6655) centre (0, 0) ccw
  arc A106 (-8.8082, 16.6655) -> (-8.8639, 16.4511) centre (-8.7381, 16.5329) ccw
  arc A107 (-9.8152, 15.9019) -> (-8.8639, 16.4511) centre (-9.325, 16.1514) ccw
  arc A108 (-9.8152, 15.9019) -> (-10.0286, 15.9609) centre (-9.9488, 15.8338) ccw
  arc A109 (-10.0286, 15.9609) -> (-10.5019, 15.6535) centre (0, 0) ccw
  arc A110 (-10.5019, 15.6535) -> (-10.5349, 15.4345) centre (-10.4184, 15.5289) ccw
  arc A111 (-11.4236, 14.7888) -> (-10.5349, 15.4345) centre (-10.9622, 15.0882) ccw
  arc A112 (-11.4236, 14.7888) -> (-11.6421, 14.8251) centre (-11.5494, 14.7072) ccw
  arc A113 (-11.6421, 14.8251) -> (-12.0807, 14.47) centre (0, 0) ccw
  arc A114 (-12.0807, 14.47) -> (-12.0905, 14.2487) centre (-11.9845, 14.3548) ccw
  arc A115 (-12.9069, 13.5137) -> (-12.0905, 14.2487) centre (-12.4793, 13.8597) ccw
  arc A116 (-12.9069, 13.5137) -> (-13.1279, 13.527) centre (-13.0235, 13.4194) ccw
  arc A117 (-13.1279, 13.527) -> (-13.527, 13.1279) centre (0, 0) ccw
  arc A118 (-13.527, 13.1279) -> (-13.5137, 12.9069) centre (-13.4194, 13.0235) ccw
  arc A119 (-14.2487, 12.0905) -> (-13.5137, 12.9069) centre (-13.8597, 12.4793) ccw
  arc A120 (-14.2487, 12.0905) -> (-14.47, 12.0807) centre (-14.3548, 11.9845) ccw
  arc A121 (-14.47, 12.0807) -> (-14.8251, 11.6421) centre (0, 0) ccw
  arc A122 (-14.8251, 11.6421) -> (-14.7888, 11.4236) centre (-14.7072, 11.5494) ccw
  arc A123 (-15.4345, 10.5349) -> (-14.7888, 11.4236) centre (-15.0882, 10.9622) ccw
  arc A124 (-15.4345, 10.5349) -> (-15.6535, 10.5019) centre (-15.5289, 10.4184) ccw
  arc A125 (-15.6535, 10.5019) -> (-15.9609, 10.0286) centre (0, 0) ccw
  arc A126 (-15.9609, 10.0286) -> (-15.9019, 9.8152) centre (-15.8338, 9.9488) ccw
  arc A127 (-16.4511, 8.8639) -> (-15.9019, 9.8152) centre (-16.1514, 9.325) ccw
  arc A128 (-16.4511, 8.8639) -> (-16.6655, 8.8082) centre (-16.5329, 8.7381) ccw
  arc A129 (-16.6655, 8.8082) -> (-16.9217, 8.3053) centre (0, 0) ccw
  arc A130 (-16.9217, 8.3053) -> (-16.8407, 8.0992) centre (-16.787, 8.2393) ccw
  arc A131 (-17.2875, 7.0957) -> (-16.8407, 8.0992) centre (-17.0376, 7.5856) ccw
  arc A132 (-17.2875, 7.0957) -> (-17.4949, 7.0179) centre (-17.3557, 6.9621) ccw
  arc A133 (-17.4949, 7.0179) -> (-17.6971, 6.491) centre (0, 0) ccw
  arc A134 (-17.6971, 6.491) -> (-17.5951, 6.2945) centre (-17.5563, 6.4394) ccw
  arc A135 (-17.9345, 5.2498) -> (-17.5951, 6.2945) centre (-17.7372, 5.7632) ccw
  arc A136 (-17.9345, 5.2498) -> (-18.1326, 5.1508) centre (-17.9883, 5.1098) ccw
  arc A137 (-18.1326, 5.1508) -> (-18.2787, 4.6056) centre (0, 0) ccw
  arc A138 (-18.2787, 4.6056) -> (-18.1566, 4.4208) centre (-18.1332, 4.569) ccw
  arc A139 (-18.385, 3.3464) -> (-18.1566, 4.4208) centre (-18.2425, 3.8776) ccw
  arc A140 (-18.385, 3.3464) -> (-18.5717, 3.2272) centre (-18.4239, 3.2015) ccw
  arc A141 (-18.5717, 3.2272) -> (-18.66, 2.6698) centre (0, 0) ccw
  arc A142 (-18.66, 2.6698) -> (-18.5193, 2.4987) centre (-18.5115, 2.6485) ccw
  arc A143 (-18.6341, 1.4063) -> (-18.5193, 2.4987) centre (-18.5478, 1.9495) ccw
  arc A144 (-18.6341, 1.4063) -> (-18.8073, 1.2682) centre (-18.6576, 1.2581) ccw
  arc A145 (-18.8073, 1.2682) -> (-18.8368, 0.7046) centre (0, 0) ccw
  arc A146 (-18.8368, 0.7046) -> (-18.679, 0.5492) centre (-18.6869, 0.699) ccw
  arc A147 (-18.679, -0.5492) -> (-18.679, 0.5492) centre (-18.65, 0) ccw
  arc A148 (-18.679, -0.5492) -> (-18.8368, -0.7046) centre (-18.6869, -0.699) ccw
  arc A149 (-18.8368, -0.7046) -> (-18.8073, -1.2682) centre (0, 0) ccw
  arc A150 (-18.8073, -1.2682) -> (-18.6341, -1.4063) centre (-18.6576, -1.2581) ccw
  arc A151 (-18.5193, -2.4987) -> (-18.6341, -1.4063) centre (-18.5478, -1.9495) ccw
  arc A152 (-18.5193, -2.4987) -> (-18.66, -2.6698) centre (-18.5115, -2.6485) ccw
  arc A153 (-18.66, -2.6698) -> (-18.5717, -3.2272) centre (0, 0) ccw
  arc A154 (-18.5717, -3.2272) -> (-18.385, -3.3464) centre (-18.4239, -3.2015) ccw
  arc A155 (-18.1566, -4.4208) -> (-18.385, -3.3464) centre (-18.2425, -3.8776) ccw
  arc A156 (-18.1566, -4.4208) -> (-18.2787, -4.6056) centre (-18.1332, -4.569) ccw
  arc A157 (-18.2787, -4.6056) -> (-18.1326, -5.1508) centre (0, 0) ccw
  arc A158 (-18.1326, -5.1508) -> (-17.9345, -5.2498) centre (-17.9883, -5.1098) ccw
  arc A159 (-17.5951, -6.2945) -> (-17.9345, -5.2498) centre (-17.7372, -5.7632) ccw
  arc A160 (-17.5951, -6.2945) -> (-17.6971, -6.491) centre (-17.5563, -6.4394) ccw
  arc A161 (-17.6971, -6.491) -> (-17.4949, -7.0179) centre (0, 0) ccw
  arc A162 (-17.4949, -7.0179) -> (-17.2875, -7.0957) centre (-17.3557, -6.9621) ccw
  arc A163 (-16.8407, -8.0992) -> (-17.2875, -7.0957) centre (-17.0376, -7.5856) ccw
  arc A164 (-16.8407, -8.0992) -> (-16.9217, -8.3053) centre (-16.787, -8.2393) ccw
  arc A165 (-16.9217, -8.3053) -> (-16.6655, -8.8082) centre (0, 0) ccw
  arc A166 (-16.6655, -8.8082) -> (-16.4511, -8.8639) centre (-16.5329, -8.7381) ccw
  arc A167 (-15.9019, -9.8152) -> (-16.4511, -8.8639) centre (-16.1514, -9.325) ccw
  arc A168 (-15.9019, -9.8152) -> (-15.9609, -10.0286) centre (-15.8338, -9.9488) ccw
  arc A169 (-15.9609, -10.0286) -> (-15.6535, -10.5019) centre (0, 0) ccw
  arc A170 (-15.6535, -10.5019) -> (-15.4345, -10.5349) centre (-15.5289, -10.4184) ccw
  arc A171 (-14.7888, -11.4236) -> (-15.4345, -10.5349) centre (-15.0882, -10.9622) ccw
  arc A172 (-14.7888, -11.4236) -> (-14.8251, -11.6421) centre (-14.7072, -11.5494) ccw
  arc A173 (-14.8251, -11.6421) -> (-14.47, -12.0807) centre (0, 0) ccw
  arc A174 (-14.47, -12.0807) -> (-14.2487, -12.0905) centre (-14.3548, -11.9845) ccw
  arc A175 (-13.5137, -12.9069) -> (-14.2487, -12.0905) centre (-13.8597, -12.4793) ccw
  arc A176 (-13.5137, -12.9069) -> (-13.527, -13.1279) centre (-13.4194, -13.0235) ccw
  arc A177 (-13.527, -13.1279) -> (-13.1279, -13.527) centre (0, 0) ccw
  arc A178 (-13.1279, -13.527) -> (-12.9069, -13.5137) centre (-13.0235, -13.4194) ccw
  arc A179 (-12.0905, -14.2487) -> (-12.9069, -13.5137) centre (-12.4793, -13.8597) ccw
  arc A180 (-12.0905, -14.2487) -> (-12.0807, -14.47) centre (-11.9845, -14.3548) ccw
  arc A181 (-12.0807, -14.47) -> (-11.6421, -14.8251) centre (0, 0) ccw
  arc A182 (-11.6421, -14.8251) -> (-11.4236, -14.7888) centre (-11.5494, -14.7072) ccw
  arc A183 (-10.5349, -15.4345) -> (-11.4236, -14.7888) centre (-10.9622, -15.0882) ccw
  arc A184 (-10.5349, -15.4345) -> (-10.5019, -15.6535) centre (-10.4184, -15.5289) ccw
  arc A185 (-10.5019, -15.6535) -> (-10.0286, -15.9609) centre (0, 0) ccw
  arc A186 (-10.0286, -15.9609) -> (-9.8152, -15.9019) centre (-9.9488, -15.8338) ccw
  arc A187 (-8.8639, -16.4511) -> (-9.8152, -15.9019) centre (-9.325, -16.1514) ccw
  arc A188 (-8.8639, -16.4511) -> (-8.8082, -16.6655) centre (-8.7381, -16.5329) ccw
  arc A189 (-8.8082, -16.6655) -> (-8.3053, -16.9217) centre (0, 0) ccw
  arc A190 (-8.3053, -16.9217) -> (-8.0992, -16.8407) centre (-8.2393, -16.787) ccw
  arc A191 (-7.0957, -17.2875) -> (-8.0992, -16.8407) centre (-7.5856, -17.0376) ccw
  arc A192 (-7.0957, -17.2875) -> (-7.0179, -17.4949) centre (-6.9621, -17.3557) ccw
  arc A193 (-7.0179, -17.4949) -> (-6.491, -17.6971) centre (0, 0) ccw
  arc A194 (-6.491, -17.6971) -> (-6.2945, -17.5951) centre (-6.4394, -17.5563) ccw
  arc A195 (-5.2498, -17.9345) -> (-6.2945, -17.5951) centre (-5.7632, -17.7372) ccw
  arc A196 (-5.2498, -17.9345) -> (-5.1508, -18.1326) centre (-5.1098, -17.9883) ccw
  arc A197 (-5.1508, -18.1326) -> (-4.6056, -18.2787) centre (0, 0) ccw
  arc A198 (-4.6056, -18.2787) -> (-4.4208, -18.1566) centre (-4.569, -18.1332) ccw
  arc A199 (-3.3464, -18.385) -> (-4.4208, -18.1566) centre (-3.8776, -18.2425) ccw
  arc A200 (-3.3464, -18.385) -> (-3.2272, -18.5717) centre (-3.2015, -18.4239) ccw
  arc A201 (-3.2272, -18.5717) -> (-2.6698, -18.66) centre (0, 0) ccw
  arc A202 (-2.6698, -18.66) -> (-2.4987, -18.5193) centre (-2.6485, -18.5115) ccw
  arc A203 (-1.4063, -18.6341) -> (-2.4987, -18.5193) centre (-1.9495, -18.5478) ccw
  arc A204 (-1.4063, -18.6341) -> (-1.2682, -18.8073) centre (-1.2581, -18.6576) ccw
  arc A205 (-1.2682, -18.8073) -> (-0.7046, -18.8368) centre (0, 0) ccw
  arc A206 (-0.7046, -18.8368) -> (-0.5492, -18.679) centre (-0.699, -18.6869) ccw
  arc A207 (0.5492, -18.679) -> (-0.5492, -18.679) centre (0, -18.65) ccw
  arc A208 (0.5492, -18.679) -> (0.7046, -18.8368) centre (0.699, -18.6869) ccw
  arc A209 (0.7046, -18.8368) -> (1.2682, -18.8073) centre (0, 0) ccw
  arc A210 (1.2682, -18.8073) -> (1.4063, -18.6341) centre (1.2581, -18.6576) ccw
  arc A211 (2.4987, -18.5193) -> (1.4063, -18.6341) centre (1.9495, -18.5478) ccw
  arc A212 (2.4987, -18.5193) -> (2.6698, -18.66) centre (2.6485, -18.5115) ccw
  arc A213 (2.6698, -18.66) -> (3.2272, -18.5717) centre (0, 0) ccw
  arc A214 (3.2272, -18.5717) -> (3.3464, -18.385) centre (3.2015, -18.4239) ccw
  arc A215 (4.4208, -18.1566) -> (3.3464, -18.385) centre (3.8776, -18.2425) ccw
  arc A216 (4.4208, -18.1566) -> (4.6056, -18.2787) centre (4.569, -18.1332) ccw
  arc A217 (4.6056, -18.2787) -> (5.1508, -18.1326) centre (0, 0) ccw
  arc A218 (5.1508, -18.1326) -> (5.2498, -17.9345) centre (5.1098, -17.9883) ccw
  arc A219 (6.2945, -17.5951) -> (5.2498, -17.9345) centre (5.7632, -17.7372) ccw
  arc A220 (6.2945, -17.5951) -> (6.491, -17.6971) centre (6.4394, -17.5563) ccw
  arc A221 (6.491, -17.6971) -> (7.0179, -17.4949) centre (0, 0) ccw
  arc A222 (7.0179, -17.4949) -> (7.0957, -17.2875) centre (6.9621, -17.3557) ccw
  arc A223 (8.0992, -16.8407) -> (7.0957, -17.2875) centre (7.5856, -17.0376) ccw
  arc A224 (8.0992, -16.8407) -> (8.3053, -16.9217) centre (8.2393, -16.787) ccw
  arc A225 (8.3053, -16.9217) -> (8.8082, -16.6655) centre (0, 0) ccw
  arc A226 (8.8082, -16.6655) -> (8.8639, -16.4511) centre (8.7381, -16.5329) ccw
  arc A227 (9.8152, -15.9019) -> (8.8639, -16.4511) centre (9.325, -16.1514) ccw
  arc A228 (9.8152, -15.9019) -> (10.0286, -15.9609) centre (9.9488, -15.8338) ccw
  arc A229 (10.0286, -15.9609) -> (10.5019, -15.6535) centre (0, 0) ccw
  arc A230 (10.5019, -15.6535) -> (10.5349, -15.4345) centre (10.4184, -15.5289) ccw
  arc A231 (11.4236, -14.7888) -> (10.5349, -15.4345) centre (10.9622, -15.0882) ccw
  arc A232 (11.4236, -14.7888) -> (11.6421, -14.8251) centre (11.5494, -14.7072) ccw
  arc A233 (11.6421, -14.8251) -> (12.0807, -14.47) centre (0, 0) ccw
  arc A234 (12.0807, -14.47) -> (12.0905, -14.2487) centre (11.9845, -14.3548) ccw
  arc A235 (12.9069, -13.5137) -> (12.0905, -14.2487) centre (12.4793, -13.8597) ccw
  arc A236 (12.9069, -13.5137) -> (13.1279, -13.527) centre (13.0235, -13.4194) ccw
  arc A237 (13.1279, -13.527) -> (13.527, -13.1279) centre (0, 0) ccw
  arc A238 (13.527, -13.1279) -> (13.5137, -12.9069) centre (13.4194, -13.0235) ccw
  arc A239 (14.2487, -12.0905) -> (13.5137, -12.9069) centre (13.8597, -12.4793) ccw
  arc A240 (14.2487, -12.0905) -> (14.47, -12.0807) centre (14.3548, -11.9845) ccw
  dimension "d58" = 40
  constraint coincident A0.centre A1.centre
  measures "d58" diameter of A0
extrude "Extrude10" add sketch "Sketch9" along normal blind 1 contours A0 | A1 A2 A3 A4 A5 A6 A7 A8 A9 A10 A11 A12 A13 A14 A15 A16 A17 A18 A19 A20 A21 A22 A23 A24 A25 A26 A27 A28 A29 A30 A31 A32 A33 A34 A35 A36 A37 A38 A39 A40 A41 A42 A43 A44 A45 A46 A47 A48 A49 A50 A51 A52 A53 A54 A55 A56 A57 A58 A59 A60 A61 A62 A63 A64 A65 A66 A67 A68 A69 A70 A71 A72 A73 A74 A75 A76 A77 A78 A79 A80 A81 A82 A83 A84 A85 A86 A87 A88 A89 A90 A91 A92 A93 A94 A95 A96 A97 A98 A99 A100 A101 A102 A103 A104 A105 A106 A107 A108 A109 A110 A111 A112 A113 A114 A115 A116 A117 A118 A119 A120 A121 A122 A123 A124 A125 A126 A127 A128 A129 A130 A131 A132 A133 A134 A135 A136 A137 A138 A139 A140 A141 A142 A143 A144 A145 A146 A147 A148 A149 A150 A151 A152 A153 A154 A155 A156 A157 A158 A159 A160 A161 A162 A163 A164 A165 A166 A167 A168 A169 A170 A171 A172 A173 A174 A175 A176 A177 A178 A179 A180 A181 A182 A183 A184 A185 A186 A187 A188 A189 A190 A191 A192 A193 A194 A195 A196 A197 A198 A199 A200 A201 A202 A203 A204 A205 A206 A207 A208 A209 A210 A211 A212 A213 A214 A215 A216 A217 A218 A219 A220 A221 A222 A223 A224 A225 A226 A227 A228 A229 A230 A231 A232 A233 A234 A235 A236 A237 A238 A239 A240
sketch "Sketch10" plane through (0, 0, 8) normal (0, 0, 1) x (-1, 0, 0)
  circle A0 centre (0, 0) radius 20
  circle A1 centre (0, 0) radius 15.5
  dimension "d66" = 31
  constraint concentric A0 A1
  measures "d66" diameter of A1
extrude "Extrude11" cut sketch "Sketch10" against normal blind 16 contours A1
extrude "Extrude12" cut 1 faces at (-18.3678, 1.7637, 8) along direction (0, 0, -1) blind 1
equation "d28 = TeethLength"
equation "d31 = ( TeethLength * 59 ) / PI"
equation "TeethLength = 2.01 mm"
